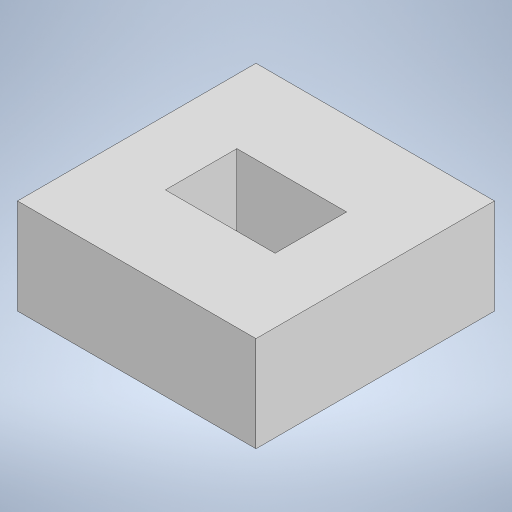
# Autodesk Inventor part: Pen_nib_stopper
Saved by Autodesk Inventor 2024 (Build 280153000, 153)
## iProperties
Created: 2025-02-15
Part Number: Pen_nib_stopper
Material: Generic
Document SubType Name: Modeling
Designer: XxPan
Density: 1 g/cm^3
Appearance: Default
Author: XxPan
Autodesk Inventor part; units mm, degrees
ref_plane "YZ Plane" through (0, 0, 0) normal (1, 0, 0) x (0, 1, 0)
ref_plane "XZ Plane" through (0, 0, 0) normal (0, 1, 0) x (-1, 0, 0)
ref_plane "XY Plane" through (0, 0, 0) normal (0, 0, 1) x (1, 0, 0)
sketch "Sketch1" plane through (0, 0, 0) normal (0, 1, 0) x (-1, 0, 0)
  line L0 (2.3, 1.5) -> (-2.3, 1.5)
  line L1 (-2.3, 1.5) -> (-2.3, -1.5)
  line L2 (-2.3, -1.5) -> (2.3, -1.5)
  line L3 (2.3, -1.5) -> (2.3, 1.5)
  line L4 (7, 0) -> (-7, 0) construction
  line L5 (0, -7) -> (0, 7) construction
  line L6 (5, 5) -> (-5, 5)
  line L7 (-5, 5) -> (-5, -5)
  line L8 (-5, -5) -> (5, -5)
  line L9 (5, -5) -> (5, 5)
  point P0 (0, 0)
  point P1 (2.3, 0)
  point P2 (0, 1.5)
  dimension "d1" = 4.6
  dimension "d2" = 3
  dimension "d3" = 10
  dimension "d4" = 10
  constraints: 16 end point, 4 parallel, 2 horizontal, 2 midpoint, 2 perpendicular, 2 point on line, 2 other
  measures "d1" distance of L2.end L1.end
  measures "d2" distance of L1.end L0.end
  measures "d3" distance of L8.end L7.end
  measures "d4" distance of L8.end L6.start
extrude "Extrusion1" add sketch "Sketch1" along normal blind 4
body "Solid1"
